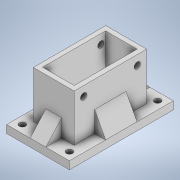
# Autodesk Inventor part: 2x1AttachmentWrap
Saved by Autodesk Inventor 2022 (Build 260153000, 153)
## iProperties
Created: 2022-02-14
Part Number: 2x1AttachmentWrap
Material: Generic
Document SubType Name: Modeling
Designer: Daniel Marquez
Density: 1 g/cm^3
Appearance: Default
Author: Daniel Marquez
Autodesk Inventor part; units mm, degrees
ref_plane "YZ Plane" through (0, 0, 0) normal (1, 0, 0) x (0, 1, 0)
ref_plane "XZ Plane" through (0, 0, 0) normal (0, 1, 0) x (-1, 0, 0)
ref_plane "XY Plane" through (0, 0, 0) normal (0, 0, 1) x (1, 0, 0)
sketch "Sketch7" plane through (0, 0, 0) normal (0, 1, 0) x (-1, 0, 0)
  line L0 (25.6032, 0) -> (25.6032, -51) construction
  line L1 (0, 3.81) -> (0, 0) construction
  line L2 (25.6032, -51) -> (0, -51) construction
  line L3 (0, -51) -> (0, 0) construction
  line L4 (0, 0) -> (25.6032, 0) construction
  line L5 (25.6032, 0) -> (25.6032, -51) construction
  line L6 (15.875, -67.51) -> (38.1, -67.51) construction
  line L7 (38.1, -15.875) -> (38.1, 16.51) projected
  line L8 (38.1, 16.51) -> (-12.7, 16.51)
  line L9 (-12.7, 16.51) -> (-12.7, -67.5132)
  line L10 (-12.7, -67.5132) -> (38.1, -67.5132)
  line L11 (38.1, -67.5132) -> (38.1, 16.51)
  line L12 (25.6032, -51) -> (0, -51)
  line L13 (0, -51) -> (0, 0)
  line L14 (0, 0) -> (25.6032, 0)
  line L15 (25.6032, 0) -> (25.6032, -51)
  dimension "d47" = 50.8
  dimension "d48" = 84.0232
  constraints: 24 end point, 6 parallel, 3 horizontal, 3 perpendicular
  measures "d47" distance of L10.end L9.end
  measures "d48" distance of L9.end L8.end
extrude "Extrusion7" add sketch "Sketch7" along normal blind 6.35
sketch "Sketch8" plane through (0, 6.35, 0) normal (0, 1, 0) x (1, 0, 0)
  line L0 (-29.21, 54.81) -> (3.81, 54.81)
  line L1 (3.81, 54.81) -> (3.81, -3.81)
  line L2 (3.81, -3.81) -> (-29.21, -3.81)
  line L3 (-29.21, -3.81) -> (-29.21, 54.81)
  line L4 (-25.6032, 0) -> (-25.6032, 51) projected
  line L5 (0, 0) -> (-25.6032, 0) projected
  line L6 (-25.6032, 51) -> (0, 51)
  line L7 (0, 51) -> (0, 0)
  line L8 (0, 0) -> (-25.6032, 0)
  line L9 (-25.6032, 0) -> (-25.6032, 51)
  dimension "d51" = 33.02
  constraints: 16 end point, 4 parallel, 2 horizontal, 2 perpendicular
  measures "d51" distance of L1.end L2.end
extrude "Extrusion8" add sketch "Sketch8" along normal blind 38.1 separate body
ref_plane "Work Plane3" through (-29.21, 6.35, -25.4) normal (0, 0, 1) x (1, 0, 0)
ref_plane "Work Plane4" through (-12.7, 6.35, 3.81) normal (1, 0, 0) x (0, 0, -1)
sketch "Sketch9" plane through (-12.7, 6.35, 3.81) normal (1, 0, 0) x (0, 0, -1)
  line L0 (3.81, 38.1) -> (54.81, 38.1) construction
  line L1 (29.31, 38.1) -> (29.31, 0) construction
  line L2 (54.81, 0) -> (3.81, 0) construction
  line L3 (-12.7, -6.35) -> (-12.7, 0) projected
  line L4 (-12.7, 0) -> (0, 14.199)
  line L5 (0, 14.199) -> (0, 0)
  line L6 (0, 0) -> (-12.7, 0)
  line L7 (71.32, 0) -> (58.62, 14.199)
  line L8 (58.62, 14.199) -> (58.62, 0)
  line L9 (58.62, 0) -> (71.32, 0)
  point P0 (3.81, -6.35)
  dimension "d56" = 19.05
  constraints: 14 end point, 3 symmetric about line, 2 midpoint, 1 perpendicular
  measures "d56" distance of L3.end L4.end
extrude "Extrusion9" add sketch "Sketch9" along normal mid plane 12.7 bodies 2
sketch "Sketch10" plane through (-29.21, 6.35, -25.4) normal (0, 0, 1) x (1, 0, 0)
  line L0 (0, 38.1) -> (33.02, 38.1) construction
  line L1 (16.51, 38.1) -> (16.4084, 0) construction
  line L2 (29.21, 0) -> (3.6068, 0) construction
  line L3 (41.91, -6.35) -> (41.91, 0) projected
  line L4 (41.91, 0) -> (33.02, 16.8485)
  line L5 (33.02, 16.8485) -> (33.02, 0)
  line L6 (33.02, 0) -> (41.91, 0)
  line L7 (-8.89, -6.35) -> (-8.89, 0) projected
  line L8 (-8.89, 0) -> (0, 16.8485)
  line L9 (0, 0) -> (0, 38.1) projected
  line L10 (0, 16.8485) -> (0, 0)
  line L11 (0, 0) -> (-8.89, 0)
  point P0 (29.21, -6.35)
  dimension "d59" = 19.05
  dimension "d60" = 19.05
  constraints: 14 end point, 2 midpoint, 2 perpendicular, 1 collinear, 1 point on line
  measures "d59" distance of L3.end L4.end
  measures "d60" distance of L7.end L8.end
extrude "Extrusion10" add sketch "Sketch10" along normal mid plane 25.4 bodies 2
sketch "Sketch11" plane through (0, 6.35, 0) normal (0, 1, 0) x (1, 0, 0)
  circle A0 centre (6.35, 61.1632) radius 2.54
  line L0 (12.7, -16.51) -> (12.7, 67.5132) projected
  line L1 (12.7, 67.5132) -> (-38.1, 67.5132) projected
  line L2 (12.7, 25.5016) -> (-38.1, 25.5016) construction
  line L3 (-38.1, 67.5132) -> (-38.1, -16.51) construction
  line L4 (-12.7, -16.51) -> (-12.7, 67.5132) construction
  circle A1 centre (6.35, -10.16) radius 2.54
  circle A2 centre (-31.75, 61.1632) radius 2.54
  circle A3 centre (-31.75, -10.16) radius 2.54
  point P0 (0, 0)
  dimension "d63" = 5.08
  dimension "d64" = 6.35
  dimension "d65" = 6.35
  constraints: 4 centre point, 4 end point, 3 midpoint, 3 symmetric about line, 3 other
  measures "d63" diameter of A0
  measures "d64" distance from line of L0 A0.centre
  measures "d65" distance from line of L1 A0.centre
extrude "Extrusion11" cut sketch "Sketch11" against normal through all bodies 1
sketch "Sketch12" plane through (-29.21, 6.35, 3.81) normal (-1, 0, 0) x (0, 0, 1)
  circle A0 centre (-51, 30.48) radius 2.54
  line L0 (-58.62, 38.1) -> (0, 38.1) construction
  line L1 (-29.31, 38.1) -> (-29.3116, -6.35) construction
  line L2 (-71.3232, -6.35) -> (12.7, -6.35) construction
  line L3 (-58.62, 0) -> (-58.62, 38.1) construction
  circle A1 centre (-7.6205, 30.4784) radius 2.54
  point P0 (-3.81, -6.35)
  dimension "d68" = 5.08
  dimension "d69" = 7.62
  dimension "d70" = 7.62
  constraints: 2 centre point, 2 end point, 2 midpoint, 1 symmetric about line, 1 other
  measures "d68" diameter of A0
  measures "d69" distance from line of L0 A0.centre
  measures "d70" distance from line of L3 A0.centre
extrude "Extrusion12" cut sketch "Sketch12" against normal through all bodies 2
body "Solid1"
body "Solid2"
body "Solid3"
